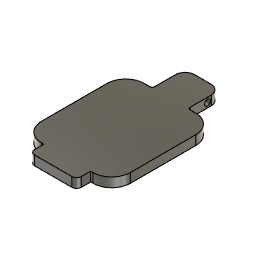
Single_Protected_Shield (Autodesk Fusion 360 design; units mm, degrees)
Autodesk Fusion 360 part; units mm, degrees
sketch "Sketch1" plane through (0, 0, 0) normal (0, 0, 1) x (1, 0, 0)
  line L0 (9.5, 29) -> (9.5, 22) construction
  line L1 (9.5, 0) -> (9.5, -3) construction
  line L2 (9.5, -3) -> (13.5, -3)
  line L3 (9.5, -3) -> (5.5, -3)
  line L4 (4.5, -2) -> (4.5, 0)
  line L5 (14.5, -2) -> (14.5, 0)
  line L6 (15, 0) -> (14.5, 0)
  line L7 (4.5, 0) -> (4, 0)
  line L8 (13.3, 22.5) -> (13.3, 27)
  line L9 (5.7, 22.5) -> (5.7, 27)
  line L10 (11.3, 29) -> (7.7, 29)
  line L11 (19, 4) -> (19, 18)
  line L12 (0, 4) -> (0, 18)
  arc A0 (0, 4) -> (4, 0) centre (4, 4) ccw
  arc A1 (15, 0) -> (19, 4) centre (15, 4) ccw
  arc A2 (19, 18) -> (15, 22) centre (15, 18) ccw
  arc A3 (4, 22) -> (0, 18) centre (4, 18) ccw
  line L13 (15, 22) -> (13.8, 22)
  arc A4 (13.3, 22.5) -> (13.8, 22) centre (13.8, 22.5) ccw
  line L14 (4, 22) -> (5.2, 22)
  arc A5 (5.2, 22) -> (5.7, 22.5) centre (5.2, 22.5) ccw
  arc A6 (13.3, 27) -> (11.3, 29) centre (11.3, 27) ccw
  arc A7 (7.7, 29) -> (5.7, 27) centre (7.7, 27) ccw
  arc A8 (13.5, -3) -> (14.5, -2) centre (13.5, -2) ccw
  arc A9 (4.5, -2) -> (5.5, -3) centre (5.5, -2) ccw
  point P0 (19, 0)
  point P1 (13.3, 22)
  dimension "d1" = 19
  dimension "d6" = 3.8
  dimension "d8" = 4
  dimension "d9" = 4
  dimension "d10" = 4
  dimension "d11" = 4
  dimension "d12" = 0.5
  dimension "d13" = 0.5
  dimension "d14" = 2
  dimension "d15" = 2
  dimension "d16" = 1
  dimension "d17" = 1
  constraint perpendicular L1 L2
  constraint perpendicular L1 L3
  constraint perpendicular L5 L6
  constraint perpendicular L9 L10
  constraint perpendicular L7 L12
  constraint tangent L7 A0
  constraint tangent L12 A0
  constraint coincident P0 L6
  constraint coincident P0 L11
  constraint tangent L6 A1
  constraint tangent L11 A1
  constraint tangent L11 A2
  constraint tangent L12 A3
  constraint tangent A3 L13
  constraint coincident P1 L8
  constraint coincident A3.start L13
  constraint tangent L8 A4
  constraint tangent L13 A4
  constraint tangent L9 A5
  constraint tangent L14 A5
  constraint tangent L10 A6
  constraint tangent L8 A6
  constraint tangent L10 A7
  constraint tangent L9 A7
  constraint tangent L5 A8
  constraint tangent L2 A8
  constraint tangent L4 A9
  constraint tangent L3 A9
  measures "d1" distance of origin P0
  measures "d6" distance of L0.end P1
  measures "d8" radius of A0
  measures "d9" radius of A1
  measures "d10" radius of A2
  measures "d11" radius of A3
  measures "d12" radius of A4
  measures "d13" radius of A5
  measures "d14" radius of A6
  measures "d15" radius of A7
  measures "d16" radius of A8
  measures "d17" radius of A9
extrude "Extrude1" add sketch "Sketch1" along normal blind 2
sketch "Sketch2" plane through (13.3, 0, 0) normal (1, 0, 0) x (0, 1, 0)
  line L0 (22.5, 0) -> (27, 0)
  line L1 (27, 0) -> (27, 2)
  line L2 (27, 2) -> (22.5, 2)
  line L3 (22.5, 2) -> (22.5, 0)
  line L4 (27, 1) -> (22.5, 1) construction
  circle A0 centre (26.2099, 1) radius 0.65
  dimension "d20" = 1.3
  constraint midpoint L1 L4.start
  constraint midpoint L3 L4.end
  constraint coincident L4 A0.centre
  measures "d20" diameter of A0
extrude "Extrude2" cut sketch "Sketch2" against normal blind 20 contours A0
